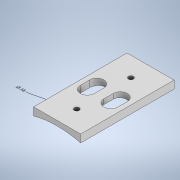
# Autodesk Inventor part: finderSupportPartV05
Saved by Autodesk Inventor 2021 (Build 250183000, 183)
## iProperties
Created: 2020-06-05
Part Number: finderSupportPartV05
Material: Generic
Document SubType Name: Modeling
Designer: robst
Density: 1 g/cm^3
Appearance: Default
Author: robst
Autodesk Inventor part; units mm, degrees
ref_plane "YZ Plane" through (0, 0, 0) normal (1, 0, 0) x (0, 1, 0)
ref_plane "XY Plane" through (0, 0, 0) normal (0, 0, 1) x (1, 0, 0)
sketch "Sketch1" plane through (0, 0, 0) normal (0, 0, 1) x (1, 0, 0)
  arc A0 (19.05, 73.7803) -> (-19.05, 73.7803) centre (0, 0) ccw
  line L0 (0, 86.4803) -> (19.05, 86.4803)
  line L1 (19.05, 86.4803) -> (19.05, 73.7803)
  line L2 (0, 76.2) -> (0, 86.4803) construction
  line L3 (0, 86.4803) -> (-19.05, 86.4803)
  line L4 (-19.05, 86.4803) -> (-19.05, 73.7803)
  dimension "d0" = 152.4
  dimension "d1" = 19.05
  dimension "d2" = 12.7
  constraints: 10 end point, 3 point on circle, 2 symmetric about line, 1 centre point, 1 coincident, 1 horizontal, 1 perpendicular, 1 vertical
  measures "d0" diameter of A0
  measures "d1" distance of L0.start L0.end
  measures "d2" distance of L0.end L1.end
extrude "Extrusion1" add sketch "Sketch1" along normal mid plane 75.6666
sketch "Sketch2" plane through (-19.05, 86.4803, 37.8333) normal (0, 1, 0) x (1, 0, 0)
  line L0 (0, 75.6666) -> (0, 0) construction
  line L1 (0, 37.8333) -> (38.1, 37.8333) construction
  line L2 (38.1, 75.6666) -> (38.1, 0) construction
  line L3 (0, 75.6666) -> (38.1, 75.6666) construction
  line L4 (19.05, 75.6666) -> (19.05, 0) construction
  line L5 (38.1, 0) -> (0, 0) construction
  line L6 (28.575, 32.4358) -> (28.575, 43.2308) construction
  line L7 (26.3525, 32.4358) -> (26.3525, 43.2308)
  line L8 (30.7975, 43.2308) -> (30.7975, 32.4358)
  arc A0 (26.3525, 32.4358) -> (30.7975, 32.4358) centre (28.575, 32.4358) ccw
  arc A1 (30.7975, 43.2308) -> (26.3525, 43.2308) centre (28.575, 43.2308) ccw
  line L9 (11.7475, 32.4358) -> (11.7475, 43.2308)
  line L10 (7.3025, 43.2308) -> (7.3025, 32.4358)
  arc A2 (7.3025, 32.4358) -> (11.7475, 32.4358) centre (9.525, 32.4358) ccw
  arc A3 (11.7475, 43.2308) -> (7.3025, 43.2308) centre (9.525, 43.2308) ccw
  point P0 (19.05, 37.8333)
  point P1 (28.575, 37.8333)
  dimension "d5" = 9.525
  dimension "d6" = 4.445
  dimension "d7" = 15.24
  dimension "d8" = 19.05
  constraints: 16 end point, 8 point on circle, 6 symmetric about line, 5 midpoint, 4 centre point, 4 tangent, 1 parallel, 1 perpendicular, 1 point on line, 2 other
  measures "d5" distance of point (28.575, 37.833) point (19.05, 37.833)
  measures "d6" distance between parallel lines of L8 L7
  measures "d8" distance of L6.end A3.centre
extrude "Extrusion2" cut sketch "Sketch2" against normal through all
ref_plane "Work Plane1" through (19.05, 73.7803, 37.8333) normal (0, 1, 0) x (-1, 0, 0)
sketch "Sketch4" plane through (19.05, 73.7803, 37.8333) normal (0, 1, 0) x (-1, 0, 0)
  line L0 (11.7475, -43.2308) -> (11.7475, -32.4358) projected
  line L1 (11.7475, -32.4358) -> (11.7475, -43.2308) construction
  line L2 (11.7475, -37.8333) -> (7.3025, -37.8333) construction
  line L3 (7.3025, -43.2308) -> (7.3025, -32.4358) construction
  line L4 (9.525, -41.6433) -> (9.525, -34.0233) construction
  line L5 (15.24, -41.6433) -> (15.24, -34.0233)
  line L6 (3.81, -34.0233) -> (3.81, -41.6433)
  arc A0 (3.81, -41.6433) -> (15.24, -41.6433) centre (9.525, -41.6433) ccw
  arc A1 (15.24, -34.0233) -> (3.81, -34.0233) centre (9.525, -34.0233) ccw
  line L7 (0, 0) -> (38.1, 0) construction
  line L8 (19.05, 0) -> (19.05, -75.6666) construction
  line L9 (38.1, -75.6666) -> (0, -75.6666) construction
  line L10 (22.86, -41.6433) -> (22.86, -34.0233)
  line L11 (34.29, -34.0233) -> (34.29, -41.6433)
  arc A2 (22.86, -41.6433) -> (34.29, -41.6433) centre (28.575, -41.6433) ccw
  arc A3 (34.29, -34.0233) -> (22.86, -34.0233) centre (28.575, -34.0233) ccw
  point P0 (19.05, -37.8333)
  point P1 (9.525, -37.8333)
  dimension "d11" = 11.43
  dimension "d12" = 19.05
  constraints: 16 end point, 8 point on circle, 6 midpoint, 6 symmetric about line, 4 centre point, 4 tangent, 1 parallel, 1 perpendicular, 2 other
  measures "d11" distance between parallel lines of L6 L5
extrude "Extrusion3" cut sketch "Sketch4" along normal blind 7.62
sketch "Sketch20" plane through (19.05, 73.7803, 37.8333) normal (1, 0, 0) x (0, 0, -1)
  line L0 (0, 12.7) -> (0, 0) projected
  line L1 (75.6666, 12.7) -> (0, 12.7) projected
  line L2 (0, 6.35) -> (75.6666, 6.35)
  line L3 (75.6666, 6.35) -> (75.6666, 12.7)
  line L4 (75.6666, 12.7) -> (0, 12.7)
  line L5 (0, 12.7) -> (0, 6.35)
  point P0 (37.8333, -73.7803)
  constraints: 8 end point, 2 parallel, 1 horizontal, 1 midpoint, 1 perpendicular
extrude "Extrusion7" cut sketch "Sketch20" against normal through all
sketch "Sketch21" plane through (19.05, 80.1303, 37.8333) normal (0, 1, 0) x (1, 0, 0)
  line L0 (-38.1, 75.6666) -> (0, 75.6666) construction
  line L1 (0, 0) -> (-38.1, 0) construction
  point P0 (-19.05, 37.8333)
  point P1 (-19.05, 59.7916)
  point P2 (-19.05, 15.875)
  dimension "d170" = 15.875
  dimension "d171" = 15.875
  measures "d170" distance from line of point (-19.05, 59.792) L0
  measures "d171" distance from line of point (-19.05, 15.875) L1
hole "Hole1" at (0, 80.1303, -21.9583) at (0, 80.1303, 21.9583) direction (0, -1, 0) diameter 3.9624 end through all thread size "10-32 UNF" class "2B" standard "ANSI Unified Screw Threads"
equation "\"d51\" = 0.125 * Sketch8_Pitch"
equation "\"Sketch8_Pitch\" = 0.79375"
equation "\"d53\" = 60deg"
equation "\"d72\" = 0.125 * Sketch10_Pitch"
equation "\"Sketch10_Pitch\" = 0.79375"
equation "\"d74\" = 60deg"
equation "\"d93\" = 0.125 * Sketch12_Pitch"
equation "\"Sketch12_Pitch\" = 0.79375"
equation "\"d95\" = 60deg"
equation "\"d114\" = 0.125 * Sketch14_Pitch"
equation "\"Sketch14_Pitch\" = 0.79375"
equation "\"d116\" = 60deg"
equation "\"d135\" = 0.125 * Sketch16_Pitch"
equation "\"Sketch16_Pitch\" = 0.79375"
equation "\"d137\" = 60deg"
equation "\"d156\" = 0.125 * Sketch18_Pitch"
equation "\"Sketch18_Pitch\" = 0.79375"
equation "\"d158\" = 60deg"
body "Solid1"
